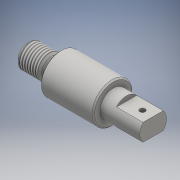
# Autodesk Inventor part: ВАЛ1
Saved by Autodesk Inventor 2016 (Build 200138000, 138)
## iProperties
Created: 2018-04-27
Part Number: ВАЛ1
Material: Типовые
Document SubType Name: Modeling
Designer: ISOB
Density: 1 g/cm^3
Appearance: По умолчанию
Author: ISOB
Autodesk Inventor part; units mm, degrees
ref_plane "YZ Plane" through (0, 0, 0) normal (1, 0, 0) x (0, 1, 0)
ref_plane "XZ Plane" through (0, 0, 0) normal (0, 1, 0) x (-1, 0, 0)
ref_plane "XY Plane" through (0, 0, 0) normal (0, 0, 1) x (1, 0, 0)
sketch "Эскиз1" plane through (0, 0, 0) normal (0, 0, 1) x (1, 0, 0)
  line L0 (0, 0) -> (0, 9)
  line L1 (0, 9) -> (17.25, 9)
  line L2 (19, 7.25) -> (17.25, 9)
  line L3 (19, 7.25) -> (23.4, 7.25)
  arc A0 (23.4, 7.25) -> (25, 8.85) centre (23.4, 8.85) ccw
  line L4 (25, 8.85) -> (25, 14)
  line L5 (25, 14) -> (26, 15)
  line L6 (26, 15) -> (64, 15)
  line L7 (65, 14) -> (64, 15)
  line L8 (65, 14) -> (65, 10)
  line L9 (65, 10) -> (75, 10)
  line L10 (75, 10) -> (75, 0)
  line L11 (0, 0) -> (75, 0)
  dimension "d0" = 9
  dimension "d1" = 17.25
  dimension "d4" = 1.75
  dimension "d5" = 1.75
  dimension "d8" = 1.6
  dimension "d9" = 23.4
  dimension "d10" = 8.85
  dimension "d11" = 5.15
  dimension "d14" = 38
  dimension "d17" = 4
  dimension "d18" = 10
  dimension "d19" = 10
  dimension "d20" = 75
  dimension "d21" = 1
  dimension "d22" = 1
  dimension "d23" = 1
  constraints: 24 end point, 3 perpendicular, 3 vertical, 2 horizontal, 2 point on circle, 1 centre point, 1 parallel
  measures "d0" distance of L0.start L0.end
  measures "d1" distance of L0.end L1.end
  measures "d4" horizontal distance of L2.start L1.end
  measures "d5" horizontal distance of L2.start L1.end
  measures "d8" radius of A0
  measures "d9" horizontal distance of L0.start A0.centre
  measures "d10" vertical distance of L0.start A0.centre
  measures "d11" distance of L4.start L4.end
  measures "d14" distance of L5.end L6.end
  measures "d17" distance of L7.start L8.end
  measures "d18" distance of L8.end L9.end
  measures "d19" distance of L9.end L10.end
  measures "d20" distance between parallel lines of L0 L10
  measures "d21" horizontal distance of L7.start L6.end
  measures "d22" horizontal distance of L7.start L6.end
  measures "d23" horizontal distance of L5.end L4.end
revolve "Вращение1" add sketch "Эскиз1" angle 360 about axis through (0, 0, 0) along (1, 0, 0)
fillet "Сопряжение1" radius 1 1 edges at (19, -7.25, 0)
thread "Резьба1" size "M18x2" class "6g" standard "ANSI Metric M Profile" full length
chamfer "Фаска1" distance 2.5 angle 45 1 edges at (0, -9, 0)
ref_plane "РабПлоскость1" through (45, 0, 0) normal (1, 0, 0) x (0, 1, 0)
sketch "Эскиз3" plane through (45, 0, 0) normal (1, 0, 0) x (0, 1, 0)
  circle A0 centre (0, 0) radius 15 projected
  circle A1 centre (0, 0) radius 14 projected
  line L0 (0, 5) -> (22.6727, 5)
  line L1 (0, 5) -> (-2.8868, 0)
  line L2 (22.6727, 0) -> (22.6727, 5)
  line L3 (-2.8868, 0) -> (22.6727, 0)
  dimension "d37" = 5
  dimension "d38" = 120
  constraints: 8 end point, 1 horizontal, 1 perpendicular
  measures "d37" distance of A1.centre L0.start
  measures "d38" angle of L0 L1
revolve "Вращение3" cut sketch "Эскиз3" angle 360 about axis through (45, -2.8868, 0) along (0, 1, 0) picked at (13.602, 4.4583) picked at (3.7044, 1.6667) contours L3 A1 L0 A0 | A0 L0 L2 L3 | L3 L1 L0 A1
sketch "Эскиз4" plane through (75, 0, 0) normal (1, 0, 0) x (0, 0, -1)
  line L0 (-6.5, 0) -> (-6.5, 7.5993)
  line L1 (-6.5, 0) -> (-6.5, -7.5993)
  line L2 (6.5, 0) -> (6.5, 7.5993)
  line L3 (6.5, 0) -> (6.5, -7.5993)
  arc A0 (6.5, 7.5993) -> (-6.5, 7.5993) centre (0, 0) ccw
  arc A1 (-6.5, -7.5993) -> (6.5, -7.5993) centre (0, 0) ccw
  dimension "d41" = 6.5
  dimension "d43" = 6.5
  constraints: 8 end point, 4 point on circle, 2 centre point, 1 coincident, 1 vertical
  measures "d41" distance of A0.centre L0.start
  measures "d43" distance of point (0, 0) L2.start
extrude "Выдавливание1" add sketch "Эскиз4" along normal blind 20
sketch "Эскиз5" plane through (75, -7.5993, -6.5) normal (0, 0, -1) x (-1, 0, 0)
  circle A0 centre (-12, 7.5993) radius 2
  point P0 (75, 7.5993)
  dimension "d47" = 4
  constraints: 1 centre point
  measures "d47" diameter of A0
extrude "Выдавливание2" cut sketch "Эскиз5" against normal blind 20
